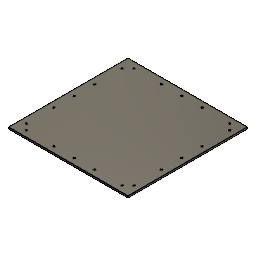
Mid_Buggy v1 v2 (Autodesk Fusion 360 design; units mm, degrees)
Autodesk Fusion 360 part; units mm, degrees
sketch "Sketch1" plane through (0, 0, 0) normal (0, 1, 0) x (1, 0, 0)
  line L0 (100, 100) -> (-100, 100)
  line L1 (-100, 100) -> (-100, -100)
  line L2 (-100, -100) -> (100, -100)
  line L3 (100, -100) -> (100, 100)
  line L4 (100, 100) -> (-100, -100) construction
  line L5 (-100, 100) -> (100, -100) construction
  circle A0 centre (90, -80) radius 1.5
  circle A1 centre (90, 0) radius 1.5
  circle A2 centre (90, 80) radius 1.5
  circle A3 centre (-90, 80) radius 1.5
  circle A4 centre (-90, 0) radius 1.5
  circle A5 centre (-90, -80) radius 1.5
  circle A6 centre (-34, -90) radius 1.5
  circle A7 centre (34, -90) radius 1.5
  circle A8 centre (-34, 90) radius 1.5
  circle A9 centre (34, 90) radius 1.5
  circle A10 centre (-90, 34) radius 1.5
  circle A11 centre (-80, 90) radius 1.5
  circle A12 centre (80, -90) radius 1.5
  circle A13 centre (90, 34) radius 1.5
  circle A14 centre (-90, -34) radius 1.5
  circle A15 centre (80, 90) radius 1.5
  circle A16 centre (0, 90) radius 1.5
  circle A17 centre (0, -90) radius 1.5
  circle A18 centre (-80, -90) radius 1.5
  circle A19 centre (90, -34) radius 1.5
  dimension "d1" = 200
  dimension "d2" = 200
  dimension "d3" = 3
  dimension "d4" = 3
  dimension "d5" = 3
  dimension "d6" = 3
  dimension "d7" = 3
  dimension "d8" = 3
  dimension "d9" = 10
  dimension "d10" = 20
  dimension "d11" = 10
  dimension "d12" = 10
  dimension "d13" = 20
  dimension "d14" = 100
  dimension "d15" = 10
  dimension "d16" = 20
  dimension "d17" = 100
  dimension "d18" = 10
  dimension "d19" = 10
  dimension "d20" = 20
  dimension "d21" = 3
  dimension "d22" = 3
  dimension "d23" = 3
  dimension "d24" = 3
  dimension "d25" = 10
  dimension "d26" = 10
  dimension "d27" = 66
  dimension "d28" = 66
  dimension "d29" = 10
  dimension "d30" = 10
  dimension "d31" = 66
  dimension "d32" = 66
  dimension "d34" = 90
  measures "d1" distance of L0.end L1.end
  measures "d2" distance of L1.end L2.end
  measures "d3" diameter of A0
  measures "d4" diameter of A1
  measures "d5" diameter of A2
  measures "d6" diameter of A3
  measures "d7" diameter of A4
  measures "d8" diameter of A5
  measures "d9" distance of L1 A5.centre
  measures "d10" distance of L2 A5.centre
  measures "d11" distance of L1 A4.centre
  measures "d12" distance of L1 A3.centre
  measures "d13" distance of L0 A3.centre
  measures "d14" distance of L0 A4.centre
  measures "d15" distance of L3 A2.centre
  measures "d16" distance of L0 A2.centre
  measures "d17" distance of L0 A1.centre
  measures "d18" distance of L3 A1.centre
  measures "d19" distance of L3 A0.centre
  measures "d20" distance of L2 A0.centre
  measures "d21" diameter of A6
  measures "d22" diameter of A7
  measures "d23" diameter of A8
  measures "d24" diameter of A9
  measures "d25" distance of L0 A8.centre
  measures "d26" distance of L0 A9.centre
  measures "d27" distance of L3 A9.centre
  measures "d28" distance of L1 A8.centre
  measures "d29" distance of L2 A6.centre
  measures "d30" distance of L2 A7.centre
  measures "d31" distance of L1 A6.centre
  measures "d32" distance of L3 A7.centre
extrude "Extrude1" add sketch "Sketch1" along normal blind 3
